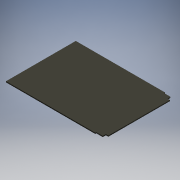
# Autodesk Inventor part: Acrylic_Panel
Saved by Autodesk Inventor 2019.4 (Build 234330000, 330)
## iProperties
Created: 2020-01-31
Part Number: Acrylic_Panel
Material: Generic
Document SubType Name: Modeling
Designer: Jorian Bruslind
Density: 1 g/cm^3
Appearance: Gunmetal
Author: Jorian Bruslind
Autodesk Inventor part; units mm, degrees
ref_plane "YZ Plane" through (0, 0, 0) normal (1, 0, 0) x (0, 1, 0)
ref_plane "XZ Plane" through (0, 0, 0) normal (0, 1, 0) x (-1, 0, 0)
ref_plane "XY Plane" through (0, 0, 0) normal (0, 0, 1) x (1, 0, 0)
sketch "Sketch1" plane through (0, 0, 0) normal (0, 1, 0) x (-1, 0, 0)
  line L0 (-240, 170.5) -> (240, 170.5)
  line L1 (240, 170.5) -> (240, -170.5)
  line L2 (240, -170.5) -> (-240, -170.5)
  line L3 (-240, -170.5) -> (-240, 170.5)
  line L4 (-240, 170.5) -> (240, -170.5) construction
  line L5 (240, 170.5) -> (-240, -170.5) construction
  point P0 (0, 0)
  dimension "d0" = 480
  dimension "d1" = 341
  constraints: 12 end point, 2 midpoint, 2 parallel, 1 horizontal, 1 perpendicular
  measures "d0" distance of L1.end L2.end
  measures "d1" distance of L0.end L1.end
extrude "Extrusion1" add sketch "Sketch1" along normal blind 5
sketch "Sketch2" plane through (0, 5, 0) normal (0, 1, 0) x (1, 0, 0)
  line L0 (240, -170.5) -> (240, 170.5) projected
  line L1 (240, -170.5) -> (240, -150.5)
  line L2 (240, -150.5) -> (228, -150.5)
  line L3 (-240, -170.5) -> (240, -170.5) projected
  line L4 (228, -170.5) -> (228, -165.5)
  line L5 (228, -170.5) -> (233, -170.5) construction
  line L6 (228, -150.5) -> (228, -165.5)
  line L7 (228, -165.5) -> (196, -165.5)
  line L8 (196, -165.5) -> (196, -170.5)
  line L9 (196, -170.5) -> (240, -170.5)
  line L10 (240, 0) -> (160.3142, 0)
  line L11 (240, 170.5) -> (240, 150.5)
  line L12 (240, 150.5) -> (228, 150.5)
  line L13 (228, 170.5) -> (228, 165.5)
  line L14 (228, 170.5) -> (233, 170.5) construction
  line L15 (228, 150.5) -> (228, 165.5)
  line L16 (228, 165.5) -> (196, 165.5)
  line L17 (196, 165.5) -> (196, 170.5)
  line L18 (196, 170.5) -> (240, 170.5)
  point P0 (0, 0)
  dimension "d4" = 20
  dimension "d5" = 12
  dimension "d6" = 5
  dimension "d7" = 90
  dimension "d8" = 15
  dimension "d9" = 32
  constraints: 34 end point, 7 symmetric about line, 5 perpendicular, 3 horizontal, 3 point on line, 1 midpoint, 1 vertical
  measures "d4" distance of L0.start L1.end
  measures "d5" distance of L1.end L2.end
  measures "d6" distance of L4.start L4.end
  measures "d7" angle of L5 L4
  measures "d8" distance of L2.end L4.end
  measures "d9" distance of L4.end L7.end
extrude "Extrusion2" cut sketch "Sketch2" against normal blind 5
body "Solid1"
